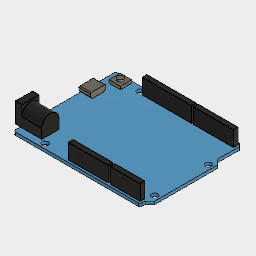
Message Panel Mount (Autodesk Fusion 360 archive; units mm, degrees)
design "2488 Adafruit Metro 328"
Autodesk Fusion 360 part; units mm, degrees
sketch "Metro-Rev-B" plane through (0, 0, 0) normal (0, 0, 1) x (1, 0, 0)
  circle A0 centre (4.318, 40.05) radius 0.35
  line L0 (65.04, 0) -> (1, 0)
  line L1 (2.118, 42) -> (2.718, 42)
  arc A1 (2.118, 34.8) -> (1.868, 34.5) centre (2.143, 34.525) ccw
  line L2 (2.718, 34.2) -> (2.118, 34.2)
  line L3 (64.516, 53.34) -> (66.04, 51.816)
  line L4 (66.04, 51.816) -> (66.04, 40.386)
  arc A2 (0, 1) -> (1, 0) centre (1, 1) ccw
  line L5 (68.58, 37.846) -> (68.58, 5.08)
  line L6 (1, 53.34) -> (64.516, 53.34)
  arc A3 (1, 53.34) -> (0, 52.34) centre (1, 52.34) ccw
  line L7 (2.718, 41.4) -> (2.118, 41.4)
  line L8 (0, 1) -> (0, 52.34)
  circle A4 centre (4.191, 17.296) radius 0.5
  circle A5 centre (4.191, 20.296) radius 0.5
  line L9 (68.58, 5.08) -> (66.04, 2.54)
  arc A6 (2.718, 34.2) -> (2.968, 34.5) centre (2.693, 34.475) ccw
  circle A7 centre (66.04, 35.56) radius 1.6
  arc A8 (2.968, 41.7) -> (2.718, 42) centre (2.693, 41.725) ccw
  circle A9 centre (15.24, 50.8) radius 1.6
  arc A10 (65.04, 0) -> (66.04, 1) centre (65.04, 1) ccw
  line L10 (2.118, 34.8) -> (2.718, 34.8)
  circle A11 centre (4.318, 36.15) radius 0.35
  arc A12 (1.868, 34.5) -> (2.118, 34.2) centre (2.143, 34.475) ccw
  circle A13 centre (13.97, 2.54) radius 1.6
  arc A14 (2.118, 42) -> (1.868, 41.7) centre (2.143, 41.725) ccw
  line L11 (66.04, 2.54) -> (66.04, 1)
  arc A15 (2.968, 34.5) -> (2.718, 34.8) centre (2.693, 34.525) ccw
  line L12 (66.04, 40.386) -> (68.58, 37.846)
  circle A16 centre (66.04, 7.62) radius 1.6
  arc A17 (2.718, 41.4) -> (2.968, 41.7) centre (2.693, 41.675) ccw
  arc A18 (1.868, 41.7) -> (2.118, 41.4) centre (2.143, 41.675) ccw
  circle A19 centre (6.4304, 7.7724) radius 0.9
  circle A20 centre (1.9304, 7.7724) radius 0.8
extrude "Extrude1" add sketch "Metro-Rev-B" along normal blind 1.64 contours A0 | L0 L3 L4 A2 L5 L6 A3 L8 L9 A10 L11 L12 | L1 L7 A8 A14 A17 A18 | A1 L2 A6 L10 A12 A15 | A4 | A5 | A11 | A19 | A20 makes body 1
sketch "headers" plane through (0, 0, 1.64) normal (0, 0, 1) x (-1, 0, 0)
  circle A0 centre (-66.04, -7.62) radius 1.6
  circle A1 centre (-66.04, -35.56) radius 1.6
  circle A2 centre (-15.24, -50.8) radius 1.6
  circle A3 centre (-13.97, -2.54) radius 1.6
  arc A4 (-1, -53.34) -> (0, -52.34) centre (-1, -52.34) ccw
  line L0 (0, -52.34) -> (0, -1)
  arc A5 (0, -1) -> (-1, 0) centre (-1, -1) ccw
  line L1 (-1, 0) -> (-65.04, 0)
  arc A6 (-65.04, 0) -> (-66.04, -1) centre (-65.04, -1) ccw
  line L2 (-66.04, -1) -> (-66.04, -2.54)
  line L3 (-66.04, -2.54) -> (-68.58, -5.08)
  line L4 (-68.58, -5.08) -> (-68.58, -37.846)
  line L5 (-68.58, -37.846) -> (-66.04, -40.386)
  line L6 (-66.04, -40.386) -> (-66.04, -51.816)
  line L7 (-66.04, -51.816) -> (-64.516, -53.34)
  line L8 (-64.516, -53.34) -> (-1, -53.34)
  line L9 (-64.94, -1.1) -> (-49.24, -1.1)
  line L10 (-49.24, -1.1) -> (-49.24, -3.6)
  line L11 (-49.24, -3.6) -> (-64.94, -3.6)
  line L12 (-64.94, -3.6) -> (-64.94, -1.1)
  line L13 (-48.24, -3.6) -> (-27.44, -3.6)
  line L14 (-27.44, -3.6) -> (-27.44, -1.1)
  line L15 (-27.44, -1.1) -> (-48.24, -1.1)
  line L16 (-48.24, -1.1) -> (-48.24, -3.6)
  line L17 (-64.94, -52.24) -> (-44.14, -52.24)
  line L18 (-44.14, -52.24) -> (-44.14, -49.74)
  line L19 (-44.14, -49.74) -> (-64.94, -49.74)
  line L20 (-64.94, -49.74) -> (-64.94, -52.24)
  line L21 (-43.14, -52.24) -> (-17.29, -52.24)
  line L22 (-17.29, -52.24) -> (-17.29, -49.74)
  line L23 (-17.29, -49.74) -> (-43.14, -49.74)
  line L24 (-43.14, -49.74) -> (-43.14, -52.24)
  dimension "d3" = 15.7
  dimension "d4" = 2.5
  dimension "d5" = 20.8
  dimension "d6" = 2.5
  dimension "d7" = 1
  dimension "d8" = 1.1
  dimension "d9" = 1.1
  dimension "d12" = 20.8
  dimension "d13" = 2.5
  dimension "d14" = 25.85
  dimension "d15" = 1.1
  dimension "d16" = 1
  dimension "d17" = 1.1
  measures "d3" distance of L9.start L9.end
  measures "d4" distance of L9.start L11.end
  measures "d5" distance of L13.start L13.end
  measures "d6" distance of L13.start L15.end
  measures "d7" distance of L10 L16
  measures "d8" distance of L1 L9
  measures "d9" distance of L2 L12
  measures "d12" distance of L17.start L17.end
  measures "d13" distance of L17.start L19.end
  measures "d14" distance of L21.start L21.end
  measures "d15" distance of L8 L17
  measures "d16" distance of L18 L24
  measures "d17" distance of L6 L20
extrude "Extrude2" add sketch "headers" along normal blind 8 separate body contours L9 L10 L11 L12 | L13 L14 L15 L16 | L17 L18 L19 L20 | L21 L22 L23 L24 makes body 2 at (59.7067, 1.1, 6.9733) makes body 3 at (34.3733, 1.1, 4.3067) makes body 4 at (25.9067, 49.74, 4.3067) makes body 5 at (51.0733, 49.74, 4.3067)
sketch "DC Jack" plane through (0, 0, 1.64) normal (0, 0, 1) x (-1, 0, 0)
  circle A0 centre (-66.04, -7.62) radius 1.6
  circle A1 centre (-66.04, -35.56) radius 1.6
  circle A2 centre (-15.24, -50.8) radius 1.6
  circle A3 centre (-13.97, -2.54) radius 1.6
  arc A4 (-1, -53.34) -> (0, -52.34) centre (-1, -52.34) ccw
  line L0 (0, -52.34) -> (0, -1)
  arc A5 (0, -1) -> (-1, 0) centre (-1, -1) ccw
  line L1 (-1, 0) -> (-65.04, 0)
  arc A6 (-65.04, 0) -> (-66.04, -1) centre (-65.04, -1) ccw
  line L2 (-66.04, -1) -> (-66.04, -2.54)
  line L3 (-66.04, -2.54) -> (-68.58, -5.08)
  line L4 (-68.58, -5.08) -> (-68.58, -37.846)
  line L5 (-68.58, -37.846) -> (-66.04, -40.386)
  line L6 (-66.04, -40.386) -> (-66.04, -51.816)
  line L7 (-66.04, -51.816) -> (-64.516, -53.34)
  line L8 (-64.516, -53.34) -> (-1, -53.34)
  line L9 (2.5, -12.5) -> (-11.25, -12.5)
  line L10 (-11.25, -12.5) -> (-11.25, -3.5)
  line L11 (-11.25, -3.5) -> (2.5, -3.5)
  line L12 (2.5, -3.5) -> (2.5, -12.5)
  line L13 (-11.25, -8) -> (2.5, -8) construction
  dimension "d18" = 3.5
  dimension "d19" = 13.75
  dimension "d20" = 2.5
  dimension "d21" = 9
  measures "d18" distance of L1 L11
  measures "d19" distance of L10.end L11.end
  measures "d20" distance of L0 L12
  measures "d21" distance of L9.end L10.end
extrude "Extrude3" add sketch "DC Jack" along normal blind 10.5 separate body contours L0 L9 L10 L11 | L0 L9 L11 L12 makes body 6
sketch "Jack Round" plane through (0, 0, 12.14) normal (0, 0, 1) x (-1, 0, 0)
  line L0 (2.5, -3.5) -> (-11.25, -3.5)
  line L1 (-11.25, -3.5) -> (-11.25, -12.5)
  line L2 (-11.25, -12.5) -> (2.5, -12.5)
  line L3 (2.5, -12.5) -> (2.5, -3.5)
  line L4 (-0.9, -12.5) -> (-0.9, -3.5)
  dimension "d24" = 3.4
  measures "d24" distance of L3 L4
extrude "Extrude4" cut sketch "Jack Round" against normal blind 1 contours L0 L1 L2 L4 bodies 6
fillet "Fillet1" radius 4.5 2 edges at (6.075, 3.5, 11.14) (6.075, 12.5, 11.14) on bodies 6
sketch "Jack Hole" plane through (-2.5, 0, 0) normal (-1, 0, 0) x (0, -1, 0)
  line L0 (-12.5, 1.64) -> (-3.5, 1.64)
  line L1 (-3.5, 1.64) -> (-3.5, 12.14)
  line L2 (-3.5, 12.14) -> (-12.5, 12.14)
  line L3 (-12.5, 12.14) -> (-12.5, 1.64)
  line L4 (-8, 12.14) -> (-8, 1.64) construction
  circle A0 centre (-8, 6.89) radius 3.5
  dimension "d28" = 7
  measures "d28" diameter of A0
extrude "Extrude5" cut sketch "Jack Hole" against normal blind 10 contours A0 bodies 6
sketch "microUSB jack" plane through (0, 0, 1.64) normal (0, 0, 1) x (-1, 0, 0)
  circle A0 centre (-66.04, -7.62) radius 1.6
  circle A1 centre (-66.04, -35.56) radius 1.6
  circle A2 centre (-15.24, -50.8) radius 1.6
  circle A3 centre (-13.97, -2.54) radius 1.6
  arc A4 (-1, -53.34) -> (0, -52.34) centre (-1, -52.34) ccw
  line L0 (0, -52.34) -> (0, -1)
  arc A5 (0, -1) -> (-1, 0) centre (-1, -1) ccw
  line L1 (-1, 0) -> (-65.04, 0)
  arc A6 (-65.04, 0) -> (-66.04, -1) centre (-65.04, -1) ccw
  line L2 (-66.04, -1) -> (-66.04, -2.54)
  line L3 (-66.04, -2.54) -> (-68.58, -5.08)
  line L4 (-68.58, -5.08) -> (-68.58, -37.846)
  line L5 (-68.58, -37.846) -> (-66.04, -40.386)
  line L6 (-66.04, -40.386) -> (-66.04, -51.816)
  line L7 (-66.04, -51.816) -> (-64.516, -53.34)
  line L8 (-64.516, -53.34) -> (-1, -53.34)
  line L9 (-6, -42.1) -> (0, -42.1)
  line L10 (0, -42.1) -> (0, -34.1)
  line L11 (0, -34.1) -> (-6, -34.1)
  line L12 (-6, -34.1) -> (-6, -42.1)
  line L13 (-6, -42.1) -> (0, -34.1) construction
  line L14 (0, -42.1) -> (-6, -34.1) construction
  point P0 (-3, -38.1)
  dimension "d31" = 38.1
  dimension "d33" = 6
  dimension "d34" = 8
  measures "d31" distance of L1 P0
  measures "d33" distance of L10.end L11.end
  measures "d34" distance of L9.start L11.end
extrude "Extrude6" add sketch "microUSB jack" along normal blind 3 separate body contours L0 L9 L10 L11 L12 makes body 7
chamfer "Chamfer1" distance 1 angle 45 2 edges at (3, 42.1, 1.64) (3, 34.1, 1.64) on bodies 7
fillet "Fillet2" radius 0.5 6 edges at (3, 42.1, 4.64) (3, 34.1, 4.64) (3, 42.1, 2.64) (3, 41.1, 1.64) (3, 34.1, 2.64) (3, 35.1, 1.64) on bodies 7
shell "Shell1" thickness 0.4 removed faces 1 at (0, 37.169, 3.64) on bodies 7
sketch "reset button" plane through (0, 0, 1.64) normal (0, 0, 1) x (-1, 0, 0)
  circle A0 centre (-66.04, -7.62) radius 1.6
  circle A1 centre (-66.04, -35.56) radius 1.6
  circle A2 centre (-15.24, -50.8) radius 1.6
  circle A3 centre (-13.97, -2.54) radius 1.6
  arc A4 (-1, -53.34) -> (0, -52.34) centre (-1, -52.34) ccw
  line L0 (0, -52.34) -> (0, -1)
  arc A5 (0, -1) -> (-1, 0) centre (-1, -1) ccw
  line L1 (-1, 0) -> (-65.04, 0)
  arc A6 (-65.04, 0) -> (-66.04, -1) centre (-65.04, -1) ccw
  line L2 (-66.04, -1) -> (-66.04, -2.54)
  line L3 (-66.04, -2.54) -> (-68.58, -5.08)
  line L4 (-68.58, -5.08) -> (-68.58, -37.846)
  line L5 (-68.58, -37.846) -> (-66.04, -40.386)
  line L6 (-66.04, -40.386) -> (-66.04, -51.816)
  line L7 (-66.04, -51.816) -> (-64.516, -53.34)
  line L8 (-64.516, -53.34) -> (-1, -53.34)
  line L9 (-9.35, -46.403) -> (-3.35, -46.403)
  line L10 (-3.35, -46.403) -> (-3.35, -52.403)
  line L11 (-3.35, -52.403) -> (-9.35, -52.403)
  line L12 (-9.35, -52.403) -> (-9.35, -46.403)
  line L13 (-9.35, -46.403) -> (-3.35, -52.403) construction
  line L14 (-3.35, -46.403) -> (-9.35, -52.403) construction
  circle A7 centre (-6.35, -49.403) radius 1.5
  point P0 (-6.35, -49.403)
  dimension "d41" = 6
  dimension "d42" = 6
  dimension "d43" = 6.35
  dimension "d44" = 49.403
  dimension "d45" = 3
  measures "d41" distance of L9.end L10.end
  measures "d42" distance of L10.end L11.end
  measures "d43" distance of L0 P0
  measures "d44" distance of L1 P0
  measures "d45" diameter of A7
extrude "Extrude7" add sketch "reset button" along normal blind 1.5 separate body contours L9 L10 L11 L12 | A7 makes body 8
extrude "Extrude8" add sketch "reset button" along normal blind 1 from surface at 1.5 contours A7 bodies 8
equation "d27 = ( 9 / 2 ) * 1 mm"
